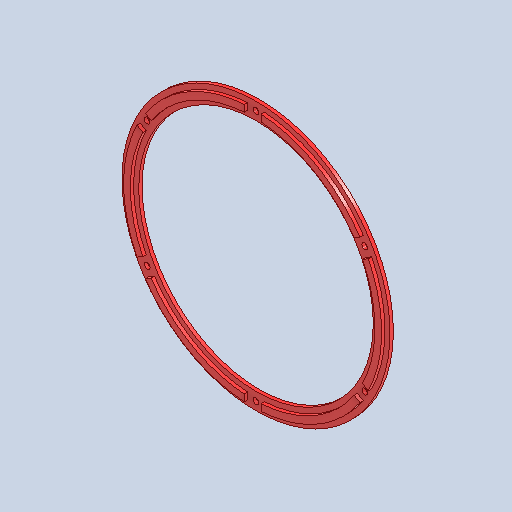
# Autodesk Inventor part: 外周ピン抑え
Saved by Autodesk Inventor 2024 (Build 280153000, 153)
## iProperties
Created: 2023-05-30
Part Number: 外周ピン抑え
Material: 一般
Document SubType Name: Modeling
Designer: yuta2
Density: 1 g/cm^3
Appearance: 淡い赤
Author: yuta2
Autodesk Inventor part; units mm, degrees
ref_plane "YZ Plane" through (0, 0, 0) normal (1, 0, 0) x (0, 1, 0)
ref_plane "XZ Plane" through (0, 0, 0) normal (0, 1, 0) x (-1, 0, 0)
ref_plane "XY Plane" through (0, 0, 0) normal (0, 0, 1) x (1, 0, 0)
sketch "スケッチ1" plane through (0, 0, 0) normal (0, 0, 1) x (1, 0, 0)
  circle A0 centre (0, 0) radius 80
  circle A1 centre (0, 0) radius 70
  dimension "d0" = 160
  dimension "d1" = 10
  constraints: 2 centre point, 1 coincident
  measures "d0" diameter of A0
  measures "d1" radial gap between concentric circles of A0 A1
extrude "押し出し1" add sketch "スケッチ1" along normal blind 2
sketch "スケッチ2" plane through (0, 0, 2) normal (0, 0, 1) x (1, 0, 0)
  point P0 (0, 0)
  point P1 (0, 75)
  dimension "d4" = 75
  constraints: 1 vertical alignment
  measures "d4" distance of point (0, 0) point (0, 75)
hole "穴1" at (0, 75, 2) direction (0, 0, -1) diameter 3.5 end through all
pattern_circular "円形状パターン1" count 6 over 360 about axis through (0, 0, 0) along (0, 0, 1) of "穴1"
sketch "スケッチ3" plane through (0, 0, 2) normal (0, 0, 1) x (1, 0, 0)
  circle A0 centre (0, 0) radius 77
  circle A1 centre (0, 0) radius 73
  dimension "d15" = 154
  dimension "d16" = 146
  constraints: 2 centre point, 2 coincident
  measures "d15" diameter of A0
  measures "d16" diameter of A1
extrude "押し出し2" add sketch "スケッチ3" along normal blind 2
sketch "スケッチ4" plane through (0, 0, 2) normal (0, 0, 1) x (1, 0, 0)
  circle A0 centre (0, 0) radius 70 projected
  circle A1 centre (0, 0) radius 80 projected
  line L0 (5, -69.8212) -> (-5, -69.8212)
  line L1 (-5, -69.8212) -> (-5, -79.8436)
  line L2 (-5, -79.8436) -> (5, -79.8436)
  line L3 (5, -79.8436) -> (5, -69.8212)
  dimension "d19" = 10
  constraints: 8 end point, 2 parallel, 2 point on circle, 1 horizontal, 1 perpendicular, 2 other
  measures "d19" distance of L0.start L0.end
extrude "押し出し3" cut sketch "スケッチ4" along normal blind 2 contours A0 L3 L2 L1
pattern_circular "円形状パターン2" count 6 over 360 about axis through (0, 0, 0) along (0, 0, 1) of "押し出し3"
equation "\"d4\" = 0.5 * D"
equation "\"D\" = 150"
